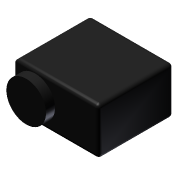
# Autodesk Inventor part: Wrist2
Saved by Autodesk Inventor 2012 (Build 160160000, 160)
## iProperties
Created: 2013-02-22
Part Number: Wrist2
Material: Default
Document SubType Name: Modeling
Designer: Andrew
Density: 1 g/cm^3
Author: Andrew
Autodesk Inventor part; units mm, degrees
ref_plane "YZ Plane" through (0, 0, 0) normal (1, 0, 0) x (0, 1, 0)
ref_plane "XZ Plane" through (0, 0, 0) normal (0, 1, 0) x (-1, 0, 0)
ref_plane "XY Plane" through (0, 0, 0) normal (0, 0, 1) x (1, 0, 0)
sketch "Sketch1" plane through (0, 0, 0) normal (0, 0, 1) x (1, 0, 0)
  line L0 (11.75, -37) -> (22.75, -37)
  line L1 (11.75, -37) -> (0.75, -37)
  line L2 (0.75, -37) -> (0.75, -32)
  line L3 (0.75, -32) -> (22.75, -32)
  line L4 (22.75, -32) -> (22.75, -37)
  line L5 (0.75, -32) -> (0.75, 6.35)
  line L6 (22.75, -32) -> (47, -32)
  line L7 (47, -32) -> (47, 6.35)
  line L8 (0.75, 6.35) -> (0.75, 9.525)
  line L9 (0.75, 9.525) -> (47, 9.525)
  line L10 (47, 9.525) -> (47, 6.35)
  point P0 (0, 0)
  dimension "d2" = 11
  dimension "d3" = 11
  dimension "d4" = 5
  constraints: 22 end point, 4 parallel, 4 perpendicular, 1 collinear
  measures "d2" distance of L0.start L0.end
  measures "d3" distance of L0.start L1.end
  measures "d4" distance of L1.end L2.end
extrude "Extrusion1" add sketch "Sketch1" along normal mid plane 26 contours L3 L5 L8 L9 L10 L7 L6
sketch "Sketch2" plane through (0.75, 9.525, 13) normal (0, 1, 0) x (1, 0, 0)
  line L0 (0, 26) -> (0, 0) projected
  line L1 (0, 13) -> (11, 13)
  circle A0 centre (11, 13) radius 10.5
  point P0 (-0.75, 13)
  dimension "d7" = 11
  dimension "d8" = 21
  constraints: 2 end point, 1 centre point, 1 coincident, 1 midpoint, 1 perpendicular
  measures "d7" distance of L1.start L1.end
  measures "d8" diameter of A0
extrude "Extrusion2" cut sketch "Sketch2" against normal blind 1
sketch "Sketch3" plane through (0.75, -32, 13) normal (0, -1, 0) x (1, 0, 0)
  line L0 (0, -26) -> (0, 0) projected
  line L1 (46.25, -26) -> (46.25, 0) projected
  line L2 (0, -13) -> (11, -13)
  circle A0 centre (11, -13) radius 11
  point P0 (-0.75, -13)
  dimension "d11" = 11
  dimension "d12" = 22
  constraints: 2 end point, 1 centre point, 1 coincident, 1 midpoint, 1 perpendicular
  measures "d11" distance of L2.start L2.end
  measures "d12" diameter of A0
extrude "Extrusion3" add sketch "Sketch3" along normal blind 5
fillet "Fillet1" radius 2 11 edges at (47, -11.2375, 13) (47, -32, 0) (47, -11.2375, -13) (47, 9.525, 0) (23.875, 9.525, 13) (23.875, -32, 13) (23.875, -32, -13) (0.75, -11.2375, 13) (0.75, 9.525, 0) (0.75, -11.2375, -13) (23.875, 9.525, -13)
body "Solid1"
